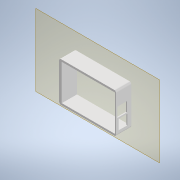
# Autodesk Inventor part: RPi Case
Saved by Autodesk Inventor 2021 (Build 250183000, 183)
## iProperties
Created: 2022-06-17
Part Number: RPi Case
Material: Generic
Document SubType Name: Modeling
Designer: cmzgt
Density: 1 g/cm^3
Appearance: Default
Author: cmzgt
Autodesk Inventor part; units mm, degrees
ref_plane "YZ Plane" through (0, 0, 0) normal (1, 0, 0) x (0, 1, 0)
ref_plane "XZ Plane" through (0, 0, 0) normal (0, 1, 0) x (-1, 0, 0)
ref_plane "XY Plane" through (0, 0, 0) normal (0, 0, 1) x (1, 0, 0)
ref_plane "Work Plane1" through (0, 0, 0) normal (0, 0, 1) x (1, 0, 0)
sketch "Sketch1" plane through (0, 0, 0) normal (0, 0, 1) x (1, 0, 0)
  line L0 (56.2342, -33.08) -> (-38.85, -33.08)
  line L1 (-38.85, -33.08) -> (-38.85, 33.08)
  line L2 (-38.85, 33.08) -> (56.2342, 33.08)
  line L3 (56.2342, 33.08) -> (56.2342, -33.08)
  line L4 (-32.5, 25) -> (-32.5, -25) projected
  line L5 (49.4242, -28) -> (-29.5, -28) projected
  line L6 (52.4242, 25) -> (52.4242, -25) projected
  line L7 (49.4242, 28) -> (-29.5, 28) projected
  line L8 (-34.405, 29.905) -> (54.3292, 29.905) projected
  line L9 (54.3292, 29.905) -> (54.3292, -29.905) projected
  line L10 (54.3292, -29.905) -> (-34.405, -29.905) projected
  line L11 (-34.405, -29.905) -> (-34.405, 29.905) projected
  line L12 (-36.31, 30.54) -> (53.6942, 30.54)
  line L13 (53.6942, 30.54) -> (53.6942, -30.54)
  line L14 (53.6942, -30.54) -> (-36.31, -30.54)
  line L15 (-36.31, -30.54) -> (-36.31, 30.54)
  point P0 (0, 0)
  dimension "d18" = 2.54
  dimension "d19" = 2.54
  dimension "d20" = 2.54
  dimension "d27" = 0.635
  dimension "d28" = 2.54
  dimension "d30" = 3.81
  dimension "d31" = 3.81
  dimension "d33" = 2.54
  constraints: 16 end point, 4 parallel, 2 horizontal, 2 perpendicular
  measures "d18" distance between parallel lines of L14 L0
  measures "d19" distance between parallel lines of L1 L15
  measures "d20" distance between parallel lines of L2 L12
  measures "d27" distance between parallel lines of L8 L12
  measures "d28" distance between parallel lines of L5 L14
  measures "d30" distance between parallel lines of L4 L15
  measures "d31" distance between parallel lines of L6 L3
  measures "d33" distance between parallel lines of L3 L13
extrude "Extrusion1" add sketch "Sketch1" along normal blind 25.4 contours L0 L1 L2 L3 | L11 L10 L13 L14 L15 L12 L8
fillet "Fillet1" radius 3.175 4 edges at (-38.85, 33.08, 12.7) (-38.85, -33.08, 12.7) (56.2342, -33.08, 12.7) (56.2342, 33.08, 12.7)
sketch "Sketch3" plane through (56.2342, -29.905, 0) normal (1, 0, 0) x (0, 0, -1)
  line L0 (-20.459, 4.3043) -> (-20.459, 20.1843) projected
  line L1 (-6.959, 4.3043) -> (-20.459, 4.3043) projected
  line L2 (-6.959, 20.1843) -> (-20.459, 20.1843) projected
  line L3 (-6.959, 4.3043) -> (-6.959, 20.1843) projected
  line L4 (-22.449, 27.9943) -> (-22.449, 33.9943) projected
  line L5 (-13.7386, 23.4443) -> (-16.7386, 23.4443) projected
  line L6 (-16.7386, 38.5443) -> (-13.7386, 38.5443) projected
  line L7 (-16.7386, 38.5443) -> (-13.7386, 38.5443) projected
  line L8 (-7.829, 30.9743) -> (-7.829, 27.9943) projected
  line L9 (-23.084, 22.8093) -> (-7.194, 22.8093)
  line L10 (-7.194, 22.8093) -> (-7.194, 39.1793)
  line L11 (-7.194, 39.1793) -> (-23.084, 39.1793)
  line L12 (-23.084, 39.1793) -> (-23.084, 22.8093)
  line L13 (-20.84, 3.9233) -> (-6.578, 3.9233)
  line L14 (-6.578, 3.9233) -> (-6.578, 20.5653)
  line L15 (-6.578, 20.5653) -> (-20.84, 20.5653)
  line L16 (-20.84, 20.5653) -> (-20.84, 3.9233)
  point P0 (0, 29.905)
  dimension "d9" = 0.635
  dimension "d10" = 0.635
  dimension "d11" = 0.635
  dimension "d12" = 0.635
  dimension "d13" = 0.381
  dimension "d14" = 0.381
  dimension "d15" = 0.381
  dimension "d16" = 0.381
  constraints: 16 end point, 4 parallel, 2 horizontal, 2 perpendicular
  measures "d9" distance between parallel lines of L6 L11
  measures "d10" distance between parallel lines of L4 L12
  measures "d11" distance between parallel lines of L5 L9
  measures "d12" distance between parallel lines of L8 L10
  measures "d13" distance between parallel lines of L2 L15
  measures "d14" distance between parallel lines of L0 L16
  measures "d15" distance between parallel lines of L1 L13
  measures "d16" distance between parallel lines of L3 L14
extrude "Extrusion2" cut sketch "Sketch3" against normal up to surface (1.905 mm away) contours L0 L2 L3 L1 | L12 L11 L10 L9 | L16 L15 L14 L13
sketch "Sketch4" plane through (0, 0, 25.4) normal (0, 0, 1) x (1, 0, 0)
  line L0 (-38.85, 29.905) -> (-38.85, -29.905) projected
  arc A0 (56.2342, 29.905) -> (53.0592, 33.08) centre (53.0592, 29.905) ccw projected
  line L1 (53.0592, 33.08) -> (-35.675, 33.08) projected
  arc A1 (-35.675, 33.08) -> (-38.85, 29.905) centre (-35.675, 29.905) ccw projected
  line L2 (-38.85, 29.905) -> (-38.85, -29.905) projected
  arc A2 (-38.85, -29.905) -> (-35.675, -33.08) centre (-35.675, -29.905) ccw projected
  line L3 (-35.675, -33.08) -> (53.0592, -33.08) projected
  arc A3 (53.0592, -33.08) -> (56.2342, -29.905) centre (53.0592, -29.905) ccw projected
  line L4 (56.2342, -29.905) -> (56.2342, 29.905) projected
  line L5 (-34.405, 29.905) -> (54.3292, 29.905) projected
  line L6 (54.3292, 29.905) -> (54.3292, -29.905) projected
  line L7 (54.3292, -29.905) -> (-34.405, -29.905) projected
  line L8 (-34.405, -29.905) -> (-34.405, 29.905) projected
  point P0 (0, 0)
extrude "Extrusion3" [suppressed]
body "Solid1"
